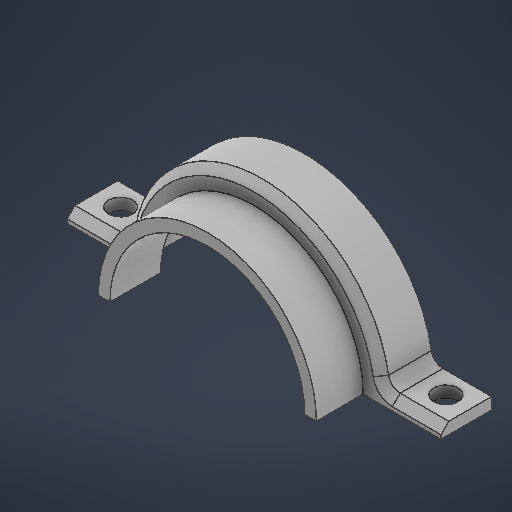
# Autodesk Inventor part: EXTRUSSOR-COUPLINGv2
Saved by Autodesk Inventor 2025.3 (Build 293356030, 356C)
## iProperties
Created: 2025-09-29
Part Number: EXTRUSSOR-COUPLINGv2
Material: Generic
Document SubType Name: Modeling
Designer: lstk1ng
Density: 1 g/cm^3
Appearance: Smooth - Medium Gray
Author: lstk1ng
Autodesk Inventor part; units mm, degrees
ref_plane "YZ Plane" through (0, 0, 0) normal (1, 0, 0) x (0, 1, 0)
ref_plane "XZ Plane" through (0, 0, 0) normal (0, 1, 0) x (-1, 0, 0)
ref_plane "XY Plane" through (0, 0, 0) normal (0, 0, 1) x (1, 0, 0)
sketch "Sketch1" plane through (0, 0, 0) normal (0, 0, 1) x (1, 0, 0)
  circle A0 centre (0, 0) radius 30
  line L0 (-33, 0) -> (-48, 0)
  line L1 (-48, 0) -> (-48, 3)
  line L2 (-48, 3) -> (-35.4965, 3)
  arc A1 (-35.4965, 3) -> (-32.5384, 5.5) centre (-35.4965, 6) ccw
  line L3 (0, 35.372) -> (0, -34.8897)
  line L4 (33, 0) -> (48, 0)
  line L5 (48, 0) -> (48, 3)
  line L6 (48, 3) -> (35.4965, 3)
  arc A2 (32.5384, 5.5) -> (35.4965, 3) centre (35.4965, 6) ccw
  arc A3 (-33, 0) -> (33, 0) centre (0, 0) ccw
  arc A4 (32.5384, 5.5) -> (-32.5384, 5.5) centre (0, 0) ccw
  line L7 (33, 0) -> (30, 0)
  line L8 (-33, 0) -> (-30, 0)
  point P0 (-32.8634, 3)
  dimension "d0" = 60
  dimension "d4" = 15
  dimension "d5" = 3
  dimension "d6" = 3
  constraints: 18 end point, 10 point on circle, 6 symmetric about line, 5 centre point, 3 horizontal, 2 coincident, 2 perpendicular, 1 point on line, 1 tangent, 1 vertical, 1 other
  measures "d0" diameter of A0
  measures "d4" distance of L0.start L0.end
  measures "d5" distance of L0.end L1.end
  measures "d6" radius of A1
extrude "Extrusion1" add sketch "Sketch1" along normal blind 13 contours A0 L3 A4 A2 L6 L5 L4 L7 | A0 L8 L0 L1 L2 A1 A4 L3
sketch "Sketch2" plane through (0, 0, 0) normal (0, 1, 0) x (-1, 0, 0)
  line L0 (-30, 0) -> (-30, 13) construction
  line L1 (-30, 0) -> (-33, 0) construction
  line L2 (-30, 0) -> (-48, 0) construction
  line L3 (-33, 0) -> (-33, 13) construction
  line L4 (-33, 13) -> (-28, 13) construction
  line L5 (-35.4965, 13) -> (-32.5384, 13) construction
  line L6 (-30, 13) -> (-28, 13)
  line L7 (-28, 13) -> (-28, 25)
  line L8 (-28, 25) -> (-25, 25)
  line L9 (-25, 25) -> (-25, 12)
  line L10 (-27, 10) -> (-30, 10)
  line L11 (-27, 10) -> (-25, 12)
  line L12 (-30, 10) -> (-30, 13)
  line L13 (0, -5) -> (0, 30) projected
  point P0 (0, 0)
  point P1 (-25, 10)
  dimension "d9" = 3
  dimension "d10" = 5
  dimension "d11" = 12
  dimension "d12" = 3
  dimension "d13" = 15
  dimension "d14" = 2
  dimension "d15" = 2
  constraints: 20 end point, 4 point on line, 3 collinear, 3 perpendicular, 2 vertical
  measures "d9" distance of L0.start L1.end
  measures "d10" distance of L3.end L4.end
  measures "d11" distance of L4.end L7.end
  measures "d12" distance of L7.end L8.end
  measures "d13" distance of L8.end point (-25, 10)
  measures "d14" distance of L10.start point (-25, 10)
  measures "d15" distance of L9.end point (-25, 10)
revolve "Revolution1" add sketch "Sketch2" angle 180 about axis through (0, 0, -10) along (0, 0, 1)
chamfer "Chamfer1" distance 2 angle 45 5 edges at (0, 33, 13) (-33.56, 3.7087, 13) (-41.7482, 3, 13) (33.56, 3.7087, 13) (41.7482, 3, 13)
sketch "Sketch3" plane through (-48, 0, 0) normal (0, -1, 0) x (1, 0, 0)
  line L0 (0, 0) -> (0, 13) construction
  line L1 (48, 0) -> (48, 25)
  line L2 (73, 25) -> (23, 25) projected
  line L3 (12.5035, 0) -> (0, 0) projected
  line L4 (6.2518, 0) -> (6.2518, 5.5) construction
  circle A0 centre (6.2518, 5.5) radius 3.1
  circle A1 centre (89.7482, 5.5) radius 3.1
  line L5 (0, 0) -> (0, 5.5) construction
  line L6 (0, 5.5) -> (6.2518, 5.5) construction
  dimension "d24" = 6.2
  dimension "d25" = 5.5
  constraints: 9 end point, 2 centre point, 2 midpoint, 1 coincident, 1 parallel, 1 perpendicular, 1 point on line, 1 symmetric about line, 1 other
  measures "d24" diameter of A0
  measures "d25" distance of L0.start L5.end
extrude "Extrusion2" cut sketch "Sketch3" against normal through all
equation "\"d15\" = d14"
body "Solid1"
